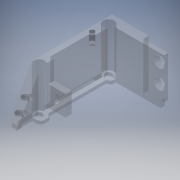
# Autodesk Inventor part: Prawybok
Saved by Autodesk Inventor 2019 (Build 230136000, 136)
## iProperties
Created: 2022-01-30
Part Number: Prawybok
Material: Tworzywo sztuczne PMMA
Document SubType Name: Modeling
Designer: Michał
Density: 1.188 g/cm^3
Appearance: Poliwęglan — przezroczysty
Mass: 7.81276 g
Surface Area: 57.7019 cm^2
Volume: 6.5764 cm^3
Author: Michał
Autodesk Inventor part; units mm, degrees
ref_plane "YZ Plane" through (0, 0, 0) normal (1, 0, 0) x (0, 1, 0)
ref_plane "XZ Plane" through (0, 0, 0) normal (0, 1, 0) x (-1, 0, 0)
ref_plane "XY Plane" through (0, 0, 0) normal (0, 0, 1) x (1, 0, 0)
sketch "Szkic1" plane through (0, 0, 0) normal (0, 1, 0) x (-1, 0, 0)
  line L0 (0, 0) -> (5, 0)
  line L1 (5, 0) -> (5, -58)
  line L2 (5, -58) -> (0, -58)
  line L3 (0, -58) -> (0, 0)
  line L4 (0, -58) -> (-14.35, -58)
  line L5 (-14.35, -58) -> (-14.35, -53)
  line L6 (-14.35, -53) -> (0, -53)
  line L7 (0, -53) -> (0, -58)
  line L8 (-14.35, -53) -> (-27.35, -53)
  line L9 (-27.35, -53) -> (-27.35, -55.2)
  line L10 (-27.35, -55.2) -> (-14.35, -55.2)
  line L11 (-14.35, -55.2) -> (-14.35, -53)
  dimension "d0" = 58
  dimension "d1" = 5
  dimension "d2" = 5
  dimension "d3" = 2.2
  dimension "d4" = 32.35
  dimension "d5" = 19.35
  constraints: 24 end point, 6 parallel, 3 horizontal, 3 perpendicular
  measures "d0" distance between parallel lines of L2 L0
  measures "d1" distance of L0.start L0.end
  measures "d2" distance between parallel lines of L4 L6
  measures "d3" distance of L8.end L9.end
  measures "d4" distance between parallel lines of L9 L1
  measures "d5" distance between parallel lines of L1 L5
extrude "Wyciągnięcie proste1" add sketch "Szkic1" along normal blind 25
sketch "Szkic2" plane through (-5, 0, -58) normal (-1, 0, 0) x (0, 0, 1)
  line L0 (58, 0) -> (5, 0) projected
  line L1 (58, 0) -> (52.8, 0)
  line L2 (52.8, 0) -> (52.8, 2)
  line L3 (52.8, 2) -> (58, 2)
  line L4 (58, 2) -> (58, 0)
  line L5 (55.6906, 2) -> (42.4115, 25)
  line L6 (42.4115, 25) -> (44.7209, 25)
  line L7 (58, 25) -> (5, 25) projected
  line L8 (58, 0) -> (58, 25) projected
  line L9 (58, 2) -> (58, 25)
  line L10 (58, 25) -> (44.7209, 25)
  line L11 (44.7209, 25) -> (58, 2) construction
  line L12 (0, 25) -> (58, 25) projected
  dimension "d8" = 2
  dimension "d9" = 2
  dimension "d10" = 5.2
  dimension "d11" = 60
  constraints: 18 end point, 3 parallel, 2 collinear, 2 perpendicular, 2 point on line, 1 horizontal
  measures "d8" distance between parallel lines of L5 L11
  measures "d9" distance between parallel lines of L0 L3
  measures "d10" distance between parallel lines of L4 L2
  measures "d11" angle of L3 L5
extrude "Wyciągnięcie proste2" cut sketch "Szkic2" against normal through all
sketch "Szkic3" plane through (0, 0, -53) normal (1, 0, 0) x (0, 0, -1)
  line L0 (-33.585, 4.5) -> (-30.585, 4.5)
  line L1 (-30.585, 4.5) -> (-30.585, 15)
  line L2 (-30.585, 15) -> (-33.585, 15)
  line L3 (-33.585, 15) -> (-33.585, 4.5)
  line L4 (-50.6906, 2) -> (-37.4115, 25) construction
  line L5 (-47.8, 0) -> (0, 0) construction
  line L6 (-33.585, 4.5) -> (-33.9517, 4.5)
  line L7 (-33.9517, 4.5) -> (-33.585, 15)
  line L8 (-33.585, 15) -> (-43.185, 15) construction
  line L9 (-37.4115, 25) -> (-50.6906, 2) construction
  point P0 (-53, 0)
  dimension "d14" = 4.5
  dimension "d16" = 3
  dimension "d17" = 88
  dimension "d29" = 10.5
  dimension "d30" = 9.6
  constraints: 14 end point, 3 horizontal, 2 parallel, 1 perpendicular, 1 point on line
  measures "d14" distance between parallel lines of L5 L0
  measures "d16" distance of L1.end L2.end
  measures "d17" angle of L7 L6
  measures "d29" distance between parallel lines of L0 L2
  measures "d30" distance of L2.end L8.end
extrude "Wyciągnięcie proste3" add sketch "Szkic3" along normal blind 9.3
sketch "Szkic4" plane through (0, 4.5, -19.0483) normal (0, 0.0348995, 0.9993908) x (1, 0, 0)
  line L0 (0, 0) -> (9.3, 0) projected
  line L1 (0, 0) -> (0, 10.5064) projected
  point P0 (0, -5.162)
  point P1 (4, 5.2)
  dimension "d20" = 5.2
  dimension "d21" = 4
  measures "d20" distance from line of L0 point (4, 5.2)
  measures "d21" distance from line of L1 point (4, 5.2)
hole "Otwór1" at (4, 9.6968, -19.2298) direction (0, -0.0348995, -0.9993908) diameter 3.4 end up to surface clearance for "Śruba ze łbem stożkowym ISO 2009/7046" size "M3" standard "ISO"
sketch "Szkic5" plane through (-5, 25, -15.5885) normal (0, 0.5, 0.8660254) x (1, 0, 0)
  line L0 (0, -26.5581) -> (5, -26.5581) construction
  line L1 (2.4, -26.5581) -> (2.4, -13.7581) construction
  line L2 (2.4, -13.7581) -> (-0.4, -13.7581) construction
  line L3 (0, -26.5581) -> (0, 0) projected
  point P0 (2.4, -20.2581)
  point P1 (0, 0)
  dimension "d32" = 6.3
  dimension "d33" = 12.8
  dimension "d41" = 2.4
  constraints: 4 end point, 1 coincident, 1 perpendicular, 1 point on line, 1 vertical, 1 other
  measures "d32" distance from line of L0 point (2.4, -20.258)
  measures "d33" distance from line of L0 point (2.4, -13.758)
  measures "d41" distance of the line from the sketch origin of L1
hole "Otwór2" at (-2.6, 13.0851, -8.7094) at (-2.6, 7.456, -5.4594) direction (0, -0.5, -0.8660254) diameter 2.459 depth 5.2 tip angle 118 thread size "M3x0.5" class "6H" standard "ISO Metric profile"
sketch "Szkic6" plane through (0, 25, 0) normal (0, 1, 0) x (1, 0, 0)
  line L0 (-5, 58) -> (-5, 15.5885) construction
  line L1 (14.35, 58) -> (-5, 58) construction
  point P0 (0, 0)
  point P1 (-1.75, 52.9)
  point P2 (-1.75, 16.3)
  dimension "d42" = 3.25
  dimension "d43" = 5.1
  dimension "d44" = 41.7
  constraints: 1 vertical alignment
  measures "d42" distance from line of L0 point (-1.75, 52.9)
  measures "d43" distance from line of L1 point (-1.75, 52.9)
  measures "d44" distance from line of L1 point (-1.75, 16.3)
hole "Otwór3" at (-1.75, 25, -52.9) at (-1.75, 25, -16.3) direction (0, -1, 0) diameter 3.4 end through all counterbore diameter 5.7 counterbore depth 23.35 clearance for "Wkręt z łbem walcowym gniazdowym ISO 4762" size "M3" standard "ISO"
sketch "Szkic8" plane through (0, 0, -5.2) normal (1, 0, 0) x (0, 0, -1)
  line L0 (8.1, 0) -> (14.1, 0)
  line L1 (14.1, 0) -> (14.1, 1.65)
  line L2 (14.1, 1.65) -> (8.1, 1.65)
  line L3 (8.1, 1.65) -> (8.1, 0)
  line L4 (44.8, 0) -> (50.8, 0)
  line L5 (50.8, 0) -> (50.8, 1.65)
  line L6 (50.8, 1.65) -> (44.8, 1.65)
  line L7 (44.8, 1.65) -> (44.8, 0)
  line L8 (0, 0) -> (47.8, 0) construction
  line L9 (13.3494, 1.65) -> (8.8506, 1.65) projected
  line L10 (49.4, 1.65) -> (46, 1.65) projected
  point P0 (-5.2, 0)
  point P1 (11.1, 1.65)
  point P2 (47.8, 1.65)
  dimension "d61" = 6
  constraints: 16 end point, 4 parallel, 3 collinear, 3 midpoint, 2 horizontal, 2 perpendicular
  measures "d61" distance of L0.start L0.end
extrude "Wyciągnięcie proste4" add sketch "Szkic8" along normal blind 2
fillet "Zaokrąglenie1" radius 2 3 edges at (2, 0.825, -13.3) (2, 0.825, -19.3) (2, 0.825, -50)
sketch "Szkic7" plane through (0, 0, -53) normal (0, 0, 1) x (1, 0, 0)
  line L0 (27.35, 0) -> (27.35, 25) projected
  line L1 (0, 0) -> (27.35, 0) projected
  line L2 (27.35, 0) -> (25.65, 0)
  line L3 (25.65, 0) -> (25.65, 3.5)
  line L4 (25.65, 3.5) -> (27.35, 3.5)
  line L5 (27.35, 3.5) -> (27.35, 0)
  point P0 (24.85, 11)
  point P1 (24.85, 21)
  dimension "d52" = 2.5
  dimension "d53" = 11
  dimension "d80" = 21
  dimension "d81" = 1.7
  dimension "d82" = 3.5
  constraints: 8 end point, 2 parallel, 1 horizontal, 1 perpendicular, 1 vertical alignment
  measures "d52" distance from line of L0 point (24.85, 11)
  measures "d53" distance from line of L1 point (24.85, 11)
  measures "d80" distance from line of L1 point (24.85, 21)
  measures "d81" distance between parallel lines of L0 L3
  measures "d82" distance between parallel lines of L1 L4
hole "Otwór4" at (24.85, 11, -53) at (24.85, 21, -53) direction (0, 0, -1) diameter 3.4 end through all countersink diameter 6.3 countersink angle 84.225 clearance for "Śruba ze łbem stożkowym ISO 2009/7046" size "M3" standard "ISO"
sketch "Szkic9" plane through (0, 1.65, -50.6506) normal (1, 0, 0) x (0, 0, -1)
  line L0 (-45.4506, -1.65) -> (-45.4506, 0.35) construction
  line L1 (2.3494, 0) -> (2.3494, -1.65) projected
  line L2 (-45.4506, 0) -> (2.3494, 0)
  line L3 (2.3494, 0) -> (2.3494, 2.2)
  line L4 (2.3494, 2.2) -> (-45.4506, 2.2)
  line L5 (-45.4506, 2.2) -> (-45.4506, 0)
  line L6 (-45.4506, -1.65) -> (-37.3506, -1.65) construction
  line L7 (-45.4506, 0) -> (-37.4506, 0)
  line L8 (-37.4506, 0) -> (-37.4506, -1.65)
  line L9 (-37.4506, -1.65) -> (-45.4506, -1.65)
  line L10 (-45.4506, -1.65) -> (-45.4506, 0)
  point P0 (-50.6506, -1.65)
  dimension "d65" = 1.65
  dimension "d66" = 2.2
  dimension "d67" = 8
  constraints: 16 end point, 4 parallel, 3 point on line, 2 horizontal, 2 perpendicular
  measures "d65" distance between parallel lines of L2 L6
  measures "d66" distance between parallel lines of L2 L4
  measures "d67" distance between parallel lines of L0 L8
extrude "Wyciągnięcie proste5" cut sketch "Szkic9" along normal blind 5 and the other way blind 2.4
sketch "Szkic11" plane through (0, 25, -18.5494) normal (1, 0, 0) x (0, 0, -1)
  line L0 (0.5254, -21.15) -> (31.5757, -21.15) projected
  line L1 (3.8655, -21.15) -> (26.0235, -21.15)
  line L2 (26.0235, -21.15) -> (26.0235, 0)
  line L3 (26.0235, 0) -> (3.8655, 0)
  line L4 (3.8655, 0) -> (3.8655, -21.15)
  line L5 (0, 0) -> (32.1011, 0) construction
  line L6 (3.8655, -20.5) -> (3.8655, -10) construction
  point P0 (-18.5494, -25)
  dimension "d85" = 22.158
  constraints: 8 end point, 2 collinear, 2 parallel, 1 horizontal, 1 perpendicular, 1 point on line
  measures "d85" distance between parallel lines of L2 L4
extrude "Wyciągnięcie proste7" cut sketch "Szkic11" against normal blind 2
sketch "Szkic10" plane through (0, 25, 0) normal (0, 1, 0) x (1, 0, 0)
  line L0 (-2.5, 45) -> (0, 45) construction
  line L1 (-2.5, 45) -> (-5, 45) construction
  line L2 (-5, 58) -> (-5, 15.5885) construction
  line L3 (0, 18.5494) -> (0, 50.6506) construction
  line L4 (14.35, 58) -> (-5, 58) construction
  circle A0 centre (-2.5, 45) radius 2.5
  point P0 (0, 0)
  dimension "d72" = 13
  dimension "d88" = 5
  constraints: 4 end point, 2 horizontal, 2 point on line, 1 centre point, 1 coincident, 1 collinear, 1 perpendicular
  measures "d72" distance from line of L4 L0.start
  measures "d88" diameter of A0
extrude "Wyciągnięcie proste6" cut sketch "Szkic7" against normal up to next
extrude "Wyciągnięcie proste8" add sketch "Szkic10" against normal blind 5
hole "Otwór5" at (-2.5, 25, -45) direction (0, -1, 0) diameter 2.459 depth 5 thread size "M3x0.5" class "6H" standard "ISO Metric profile"
